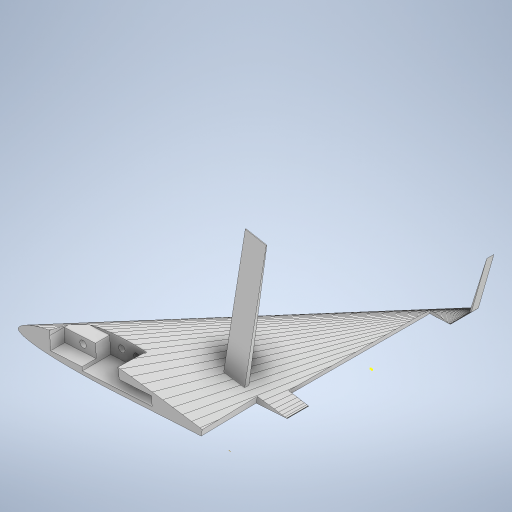
# Autodesk Inventor part: Część3
Saved by Autodesk Inventor 2023 (Build 270158000, 158)
## iProperties
Created: 2024-01-30
Part Number: Część3
Material: Ogólny
Document SubType Name: Modeling
Designer: domin
Density: 1 g/cm^3
Appearance: Domyślna
Author: domin
Autodesk Inventor part; units mm, degrees
ref_plane "YZ Plane" through (0, 0, 0) normal (1, 0, 0) x (0, 1, 0)
sketch "Szkic1" plane through (0, 0, 0) normal (0, 0, 1) x (1, 0, 0)
  line L0 (1, 0) -> (0.99647, 0.00045)
  line L1 (0.99647, 0.00045) -> (0.98625, 0.00202)
  line L2 (0.98625, 0.00202) -> (0.97011, 0.00489)
  line L3 (0.97011, 0.00489) -> (0.9487, 0.00881)
  line L4 (0.9487, 0.00881) -> (0.92238, 0.01337)
  line L5 (0.92238, 0.01337) -> (0.89128, 0.01841)
  line L6 (0.89128, 0.01841) -> (0.85576, 0.024)
  line L7 (0.85576, 0.024) -> (0.81633, 0.03011)
  line L8 (0.81633, 0.03011) -> (0.77357, 0.03666)
  line L9 (0.77357, 0.03666) -> (0.72806, 0.04352)
  line L10 (0.72806, 0.04352) -> (0.68043, 0.05055)
  line L11 (0.68043, 0.05055) -> (0.63132, 0.05759)
  line L12 (0.63132, 0.05759) -> (0.58139, 0.06441)
  line L13 (0.58139, 0.06441) -> (0.53129, 0.07079)
  line L14 (0.53129, 0.07079) -> (0.48169, 0.07638)
  line L15 (0.48169, 0.07638) -> (0.43306, 0.08075)
  line L16 (0.43306, 0.08075) -> (0.38567, 0.08362)
  line L17 (0.38567, 0.08362) -> (0.33981, 0.08483)
  line L18 (0.33981, 0.08483) -> (0.29573, 0.0843)
  line L19 (0.29573, 0.0843) -> (0.25363, 0.08205)
  line L20 (0.25363, 0.08205) -> (0.21371, 0.07819)
  line L21 (0.21371, 0.07819) -> (0.17625, 0.073)
  line L22 (0.17625, 0.073) -> (0.14162, 0.06669)
  line L23 (0.14162, 0.06669) -> (0.11018, 0.05944)
  line L24 (0.11018, 0.05944) -> (0.08225, 0.05143)
  line L25 (0.08225, 0.05143) -> (0.05808, 0.04282)
  line L26 (0.05808, 0.04282) -> (0.03791, 0.03383)
  line L27 (0.03791, 0.03383) -> (0.02189, 0.02468)
  line L28 (0.02189, 0.02468) -> (0.01015, 0.01565)
  line L29 (0.01015, 0.01565) -> (0.00279, 0.00714)
  line L30 (0.00279, 0.00714) -> (0, -0.00015)
  line L31 (0, -0.00015) -> (0.00304, -0.00626)
  line L32 (0.00304, -0.00626) -> (0.01212, -0.01204)
  line L33 (0.01212, -0.01204) -> (0.02628, -0.0175)
  line L34 (0.02628, -0.0175) -> (0.04543, -0.02234)
  line L35 (0.04543, -0.02234) -> (0.06943, -0.02649)
  line L36 (0.06943, -0.02649) -> (0.09807, -0.02991)
  line L37 (0.09807, -0.02991) -> (0.13109, -0.03257)
  line L38 (0.13109, -0.03257) -> (0.16817, -0.03448)
  line L39 (0.16817, -0.03448) -> (0.20893, -0.03565)
  line L40 (0.20893, -0.03565) -> (0.25292, -0.03611)
  line L41 (0.25292, -0.03611) -> (0.29966, -0.03586)
  line L42 (0.29966, -0.03586) -> (0.34861, -0.03487)
  line L43 (0.34861, -0.03487) -> (0.39937, -0.03302)
  line L44 (0.39937, -0.03302) -> (0.45165, -0.03044)
  line L45 (0.45165, -0.03044) -> (0.50495, -0.02744)
  line L46 (0.50495, -0.02744) -> (0.5586, -0.02425)
  line L47 (0.5586, -0.02425) -> (0.61189, -0.02102)
  line L48 (0.61189, -0.02102) -> (0.66414, -0.01787)
  line L49 (0.66414, -0.01787) -> (0.71467, -0.01488)
  line L50 (0.71467, -0.01488) -> (0.76283, -0.01212)
  line L51 (0.76283, -0.01212) -> (0.80796, -0.00963)
  line L52 (0.80796, -0.00963) -> (0.84948, -0.00744)
  line L53 (0.84948, -0.00744) -> (0.88681, -0.00555)
  line L54 (0.88681, -0.00555) -> (0.91942, -0.0039)
  line L55 (0.91942, -0.0039) -> (0.94699, -0.00239)
  line L56 (0.94699, -0.00239) -> (0.9693, -0.00108)
  line L57 (0.9693, -0.00108) -> (0.98598, -0.00026)
  line L58 (0.98598, -0.00026) -> (0.99643, 0)
  line L59 (0.99643, 0) -> (1, 0)
  point P0 (0, 0)
  dimension "d0" = 7.26481
  dimension "d1" = 178.531
  dimension "d2" = 8.69006
  dimension "d3" = 177.182
  dimension "d4" = 169.921
  dimension "d5" = 176.889
  dimension "d6" = 169.375
  dimension "d7" = 2.56425
  dimension "d8" = 169.6
  dimension "d9" = 1.94039
  dimension "d10" = 10.1614
  dimension "d11" = 1.67882
  dimension "d12" = 10.1632
  dimension "d13" = 1.54358
  dimension "d14" = 169.716
  dimension "d15" = 1.44409
  dimension "d16" = 169.577
  dimension "d17" = 1.3072
  dimension "d18" = 169.455
  dimension "d19" = 1.1312
  dimension "d20" = 169.349
  dimension "d21" = 0.89306
  dimension "d22" = 169.285
  dimension "d23" = 0.51316
  dimension "d24" = 169.267
  dimension "d25" = 0.00752
  dimension "d26" = 169.332
  dimension "d27" = 0.83462
  dimension "d28" = 169.514
  dimension "d29" = 2.12988
  dimension "d30" = 10.09
  dimension "d31" = 3.79914
  dimension "d32" = 9.35209
  dimension "d33" = 5.75343
  dimension "d34" = 8.42344
  dimension "d35" = 172.046
  dimension "d36" = 7.57127
  dimension "d37" = 169.676
  dimension "d38" = 167.212
  dimension "d39" = 6.6657
  dimension "d40" = 164.847
  dimension "d41" = 5.62061
  dimension "d42" = 162.409
  dimension "d43" = 4.3161
  dimension "d44" = 159.75
  dimension "d45" = 2.65917
  dimension "d46" = 156.733
  dimension "d47" = 0.45517
  dimension "d48" = 153.128
  dimension "d49" = 2.54557
  dimension "d50" = 148.712
  dimension "d51" = 6.91918
  dimension "d52" = 143.002
  dimension "d53" = 13.8215
  dimension "d54" = 135.169
  dimension "d55" = 25.2145
  dimension "d56" = 123.591
  dimension "d57" = 56.2828
  dimension "d58" = 103.678
  dimension "d59" = 0.12646
  dimension "d60" = 0
  dimension "d61" = 0.15175
  dimension "d62" = 0.02478
  dimension "d63" = 0.17465
  constraints: 120 end point, 1 horizontal
  measures "d0" angle of L0 L59
  measures "d1" angle of L0 L1
  measures "d2" angle of L0 L58
  measures "d3" angle of L0 L2
  measures "d4" angle of L0 L57
  measures "d5" angle of L0 L3
  measures "d6" angle of L0 L56
  measures "d7" angle of L0 L4
  measures "d8" angle of L0 L55
  measures "d9" angle of L0 L5
  measures "d10" angle of L0 L54
  measures "d11" angle of L0 L6
  measures "d12" angle of L0 L53
  measures "d13" angle of L0 L7
  measures "d14" angle of L0 L52
  measures "d15" angle of L0 L8
  measures "d16" angle of L0 L51
  measures "d17" angle of L0 L9
  measures "d18" angle of L0 L50
  measures "d19" angle of L0 L10
  measures "d20" angle of L0 L49
  measures "d21" angle of L0 L11
  measures "d22" angle of L0 L48
  measures "d23" angle of L0 L12
  measures "d24" angle of L0 L47
  measures "d25" angle of L0 L13
  measures "d26" angle of L0 L46
  measures "d27" angle of L0 L14
  measures "d28" angle of L0 L45
  measures "d29" angle of L0 L15
  measures "d30" angle of L0 L44
  measures "d31" angle of L0 L16
  measures "d32" angle of L0 L43
  measures "d33" angle of L0 L17
  measures "d34" angle of L0 L42
  measures "d35" angle of L0 L18
  measures "d36" angle of L0 L41
  measures "d37" angle of L0 L19
  measures "d38" angle of L0 L20
  measures "d39" angle of L0 L40
  measures "d40" angle of L0 L21
  measures "d41" angle of L0 L39
  measures "d42" angle of L0 L22
  measures "d43" angle of L0 L38
  measures "d44" angle of L0 L23
  measures "d45" angle of L0 L37
  measures "d46" angle of L0 L24
  measures "d47" angle of L0 L36
  measures "d48" angle of L0 L25
  measures "d49" angle of L0 L35
  measures "d50" angle of L0 L26
  measures "d51" angle of L0 L34
  measures "d52" angle of L0 L27
  measures "d53" angle of L0 L33
  measures "d54" angle of L0 L28
  measures "d55" angle of L0 L32
  measures "d56" angle of L0 L29
  measures "d57" angle of L0 L31
  measures "d58" angle of L0 L30
  measures "d59" distance from line of point (0, 0) L0
  measures "d60" distance from line of point (0, 0) L59
  measures "d61" distance from line of point (0, 0) L1
  measures "d62" distance from line of point (0, 0) L58
  measures "d63" distance from line of point (0, 0) L2
ref_plane "Płaszczyzna konstrukcyjna2" through (0, 0, 175) normal (0, 0, 1) x (1, 0, 0)
sketch "Szkic6" plane through (0, 0, 175) normal (0, 0, 1) x (1, 0, 0)
  line L0 (1, 0) -> (0.4705, 0.0675)
  line L1 (0.4705, 0.0675) -> (-1.0625, 0.303)
  line L2 (-1.0625, 0.303) -> (-3.4835, 0.7335)
  line L3 (-3.4835, 0.7335) -> (-6.695, 1.3215)
  line L4 (-6.695, 1.3215) -> (-10.643, 2.0055)
  line L5 (-10.643, 2.0055) -> (-15.308, 2.7615)
  line L6 (-15.308, 2.7615) -> (-20.636, 3.6)
  line L7 (-20.636, 3.6) -> (-26.5505, 4.5165)
  line L8 (-26.5505, 4.5165) -> (-32.9645, 5.499)
  line L9 (-32.9645, 5.499) -> (-39.791, 6.528)
  line L10 (-39.791, 6.528) -> (-46.9355, 7.5825)
  line L11 (-46.9355, 7.5825) -> (-54.302, 8.6385)
  line L12 (-54.302, 8.6385) -> (-61.7915, 9.6615)
  line L13 (-61.7915, 9.6615) -> (-69.3065, 10.6185)
  line L14 (-69.3065, 10.6185) -> (-76.7465, 11.457)
  line L15 (-76.7465, 11.457) -> (-84.041, 12.1125)
  line L16 (-84.041, 12.1125) -> (-91.1495, 12.543)
  line L17 (-91.1495, 12.543) -> (-98.0285, 12.7245)
  line L18 (-98.0285, 12.7245) -> (-104.6405, 12.645)
  line L19 (-104.6405, 12.645) -> (-110.9555, 12.3075)
  line L20 (-110.9555, 12.3075) -> (-116.9435, 11.7285)
  line L21 (-116.9435, 11.7285) -> (-122.5625, 10.95)
  line L22 (-122.5625, 10.95) -> (-127.757, 10.0035)
  line L23 (-127.757, 10.0035) -> (-132.473, 8.916)
  line L24 (-132.473, 8.916) -> (-136.6625, 7.7145)
  line L25 (-136.6625, 7.7145) -> (-140.288, 6.423)
  line L26 (-140.288, 6.423) -> (-143.3135, 5.0745)
  line L27 (-143.3135, 5.0745) -> (-145.7165, 3.702)
  line L28 (-145.7165, 3.702) -> (-147.4775, 2.3475)
  line L29 (-147.4775, 2.3475) -> (-148.5815, 1.071)
  line L30 (-148.5815, 1.071) -> (-149, -0.0225)
  line L31 (-149, -0.0225) -> (-148.544, -0.939)
  line L32 (-148.544, -0.939) -> (-147.182, -1.806)
  line L33 (-147.182, -1.806) -> (-145.058, -2.625)
  line L34 (-145.058, -2.625) -> (-142.1855, -3.351)
  line L35 (-142.1855, -3.351) -> (-138.5855, -3.9735)
  line L36 (-138.5855, -3.9735) -> (-134.2895, -4.4865)
  line L37 (-134.2895, -4.4865) -> (-129.3365, -4.8855)
  line L38 (-129.3365, -4.8855) -> (-123.7745, -5.172)
  line L39 (-123.7745, -5.172) -> (-117.6605, -5.3475)
  line L40 (-117.6605, -5.3475) -> (-111.062, -5.4165)
  line L41 (-111.062, -5.4165) -> (-104.051, -5.379)
  line L42 (-104.051, -5.379) -> (-96.7085, -5.2305)
  line L43 (-96.7085, -5.2305) -> (-89.0945, -4.953)
  line L44 (-89.0945, -4.953) -> (-81.2525, -4.566)
  line L45 (-81.2525, -4.566) -> (-73.2575, -4.116)
  line L46 (-73.2575, -4.116) -> (-65.21, -3.6375)
  line L47 (-65.21, -3.6375) -> (-57.2165, -3.153)
  line L48 (-57.2165, -3.153) -> (-49.379, -2.6805)
  line L49 (-49.379, -2.6805) -> (-41.7995, -2.232)
  line L50 (-41.7995, -2.232) -> (-34.5755, -1.818)
  line L51 (-34.5755, -1.818) -> (-27.806, -1.4445)
  line L52 (-27.806, -1.4445) -> (-21.578, -1.116)
  line L53 (-21.578, -1.116) -> (-15.9785, -0.8325)
  line L54 (-15.9785, -0.8325) -> (-11.087, -0.585)
  line L55 (-11.087, -0.585) -> (-6.9515, -0.3585)
  line L56 (-6.9515, -0.3585) -> (-3.605, -0.162)
  line L57 (-3.605, -0.162) -> (-1.103, -0.039)
  line L58 (-1.103, -0.039) -> (0.4645, 0)
  line L59 (0.4645, 0) -> (1, 0)
  point P0 (0, 0)
  dimension "d367" = 7.26481
  dimension "d368" = 178.531
  dimension "d369" = 8.69006
  dimension "d370" = 177.182
  dimension "d371" = 169.921
  dimension "d372" = 176.889
  dimension "d373" = 169.375
  dimension "d374" = 2.56425
  dimension "d375" = 169.6
  dimension "d376" = 1.94039
  dimension "d377" = 10.1614
  dimension "d378" = 1.67882
  dimension "d379" = 10.1632
  dimension "d380" = 1.54358
  dimension "d381" = 169.716
  dimension "d382" = 1.44409
  dimension "d383" = 169.577
  dimension "d384" = 1.3072
  dimension "d385" = 169.455
  dimension "d386" = 1.1312
  dimension "d387" = 169.349
  dimension "d388" = 0.89306
  dimension "d389" = 169.285
  dimension "d390" = 0.51316
  dimension "d391" = 169.267
  dimension "d392" = 0.00752
  dimension "d393" = 169.332
  dimension "d394" = 0.83462
  dimension "d395" = 169.514
  dimension "d396" = 2.12988
  dimension "d397" = 10.09
  dimension "d398" = 3.79914
  dimension "d399" = 9.35209
  dimension "d400" = 5.75343
  dimension "d401" = 8.42344
  dimension "d402" = 172.046
  dimension "d403" = 7.57127
  dimension "d404" = 169.676
  dimension "d405" = 167.212
  dimension "d406" = 6.6657
  dimension "d407" = 164.847
  dimension "d408" = 5.62061
  dimension "d409" = 162.409
  dimension "d410" = 4.3161
  dimension "d411" = 159.75
  dimension "d412" = 2.65917
  dimension "d413" = 156.733
  dimension "d414" = 0.45517
  dimension "d415" = 153.128
  dimension "d416" = 2.54557
  dimension "d417" = 148.712
  dimension "d418" = 6.91918
  dimension "d419" = 143.002
  dimension "d420" = 13.8215
  dimension "d421" = 135.169
  dimension "d422" = 25.2145
  dimension "d423" = 123.591
  dimension "d424" = 56.2828
  dimension "d425" = 103.678
  dimension "d426" = 0.12646
  dimension "d427" = 0
  dimension "d428" = 0.13816
  dimension "d429" = 0.01155
  dimension "d430" = 0.11231
  constraints: 120 end point, 1 horizontal
  measures "d367" angle of L0 L59
  measures "d368" angle of L0 L1
  measures "d369" angle of L0 L58
  measures "d370" angle of L0 L2
  measures "d371" angle of L0 L57
  measures "d372" angle of L0 L3
  measures "d373" angle of L0 L56
  measures "d374" angle of L0 L4
  measures "d375" angle of L0 L55
  measures "d376" angle of L0 L5
  measures "d377" angle of L0 L54
  measures "d378" angle of L0 L6
  measures "d379" angle of L0 L53
  measures "d380" angle of L0 L7
  measures "d381" angle of L0 L52
  measures "d382" angle of L0 L8
  measures "d383" angle of L0 L51
  measures "d384" angle of L0 L9
  measures "d385" angle of L0 L50
  measures "d386" angle of L0 L10
  measures "d387" angle of L0 L49
  measures "d388" angle of L0 L11
  measures "d389" angle of L0 L48
  measures "d390" angle of L0 L12
  measures "d391" angle of L0 L47
  measures "d392" angle of L0 L13
  measures "d393" angle of L0 L46
  measures "d394" angle of L0 L14
  measures "d395" angle of L0 L45
  measures "d396" angle of L0 L15
  measures "d397" angle of L0 L44
  measures "d398" angle of L0 L16
  measures "d399" angle of L0 L43
  measures "d400" angle of L0 L17
  measures "d401" angle of L0 L42
  measures "d402" angle of L0 L18
  measures "d403" angle of L0 L41
  measures "d404" angle of L0 L19
  measures "d405" angle of L0 L20
  measures "d406" angle of L0 L40
  measures "d407" angle of L0 L21
  measures "d408" angle of L0 L39
  measures "d409" angle of L0 L22
  measures "d410" angle of L0 L38
  measures "d411" angle of L0 L23
  measures "d412" angle of L0 L37
  measures "d413" angle of L0 L24
  measures "d414" angle of L0 L36
  measures "d415" angle of L0 L25
  measures "d416" angle of L0 L35
  measures "d417" angle of L0 L26
  measures "d418" angle of L0 L34
  measures "d419" angle of L0 L27
  measures "d420" angle of L0 L33
  measures "d421" angle of L0 L28
  measures "d422" angle of L0 L32
  measures "d423" angle of L0 L29
  measures "d424" angle of L0 L31
  measures "d425" angle of L0 L30
  measures "d426" distance from line of point (0, 0) L0
  measures "d427" distance from line of point (0, 0) L59
  measures "d428" distance from line of point (0, 0) L1
  measures "d429" distance from line of point (0, 0) L58
  measures "d430" distance from line of point (0, 0) L2
sketch "Szkic1 outline for Wyciągnięcie złożone2" plane through (0, 0, 0) normal (0, 0, 1) x (1, 0, 0)
  line L0 (0.98598, -0.00026) -> (0.99647, 0.00045)
  line L1 (0.9693, -0.00108) -> (0.98598, -0.00026)
  line L2 (0.94699, -0.00239) -> (0.9693, -0.00108)
  line L3 (0.91942, -0.0039) -> (0.94699, -0.00239)
  line L4 (0.88681, -0.00555) -> (0.91942, -0.0039)
  line L5 (0.84948, -0.00744) -> (0.88681, -0.00555)
  line L6 (0.80796, -0.00963) -> (0.84948, -0.00744)
  line L7 (0.76283, -0.01212) -> (0.80796, -0.00963)
  line L8 (0.71467, -0.01488) -> (0.76283, -0.01212)
  line L9 (0.66414, -0.01787) -> (0.71467, -0.01488)
  line L10 (0.61189, -0.02102) -> (0.66414, -0.01787)
  line L11 (0.5586, -0.02425) -> (0.61189, -0.02102)
  line L12 (0.50495, -0.02744) -> (0.5586, -0.02425)
  line L13 (0.45165, -0.03044) -> (0.50495, -0.02744)
  line L14 (0.39937, -0.03302) -> (0.45165, -0.03044)
  line L15 (0.34861, -0.03487) -> (0.39937, -0.03302)
  line L16 (0.29966, -0.03586) -> (0.34861, -0.03487)
  line L17 (0.25292, -0.03611) -> (0.29966, -0.03586)
  line L18 (0.20893, -0.03565) -> (0.25292, -0.03611)
  line L19 (0.16817, -0.03448) -> (0.20893, -0.03565)
  line L20 (0.13109, -0.03257) -> (0.16817, -0.03448)
  line L21 (0.09807, -0.02991) -> (0.13109, -0.03257)
  line L22 (0.06943, -0.02649) -> (0.09807, -0.02991)
  line L23 (0.04543, -0.02234) -> (0.06943, -0.02649)
  line L24 (0.02628, -0.0175) -> (0.04543, -0.02234)
  line L25 (0.01212, -0.01204) -> (0.02628, -0.0175)
  line L26 (0.00304, -0.00626) -> (0.01212, -0.01204)
  line L27 (0, -0.00015) -> (0.00304, -0.00626)
  line L28 (0.00279, 0.00714) -> (0, -0.00015)
  line L29 (0.01015, 0.01565) -> (0.00279, 0.00714)
  line L30 (0.02189, 0.02468) -> (0.01015, 0.01565)
  line L31 (0.03791, 0.03383) -> (0.02189, 0.02468)
  line L32 (0.05808, 0.04282) -> (0.03791, 0.03383)
  line L33 (0.08225, 0.05143) -> (0.05808, 0.04282)
  line L34 (0.11018, 0.05944) -> (0.08225, 0.05143)
  line L35 (0.14162, 0.06669) -> (0.11018, 0.05944)
  line L36 (0.17625, 0.073) -> (0.14162, 0.06669)
  line L37 (0.21371, 0.07819) -> (0.17625, 0.073)
  line L38 (0.25363, 0.08205) -> (0.21371, 0.07819)
  line L39 (0.29573, 0.0843) -> (0.25363, 0.08205)
  line L40 (0.33981, 0.08483) -> (0.29573, 0.0843)
  line L41 (0.38567, 0.08362) -> (0.33981, 0.08483)
  line L42 (0.43306, 0.08075) -> (0.38567, 0.08362)
  line L43 (0.48169, 0.07638) -> (0.43306, 0.08075)
  line L44 (0.53129, 0.07079) -> (0.48169, 0.07638)
  line L45 (0.58139, 0.06441) -> (0.53129, 0.07079)
  line L46 (0.63132, 0.05759) -> (0.58139, 0.06441)
  line L47 (0.68043, 0.05055) -> (0.63132, 0.05759)
  line L48 (0.72806, 0.04352) -> (0.68043, 0.05055)
  line L49 (0.77357, 0.03666) -> (0.72806, 0.04352)
  line L50 (0.81633, 0.03011) -> (0.77357, 0.03666)
  line L51 (0.85576, 0.024) -> (0.81633, 0.03011)
  line L52 (0.89128, 0.01841) -> (0.85576, 0.024)
  line L53 (0.92238, 0.01337) -> (0.89128, 0.01841)
  line L54 (0.9487, 0.00881) -> (0.92238, 0.01337)
  line L55 (0.97011, 0.00489) -> (0.9487, 0.00881)
  line L56 (0.98625, 0.00202) -> (0.97011, 0.00489)
  line L57 (0.99647, 0.00045) -> (0.98625, 0.00202)
sketch "Szkic6 outline for Wyciągnięcie złożone2" plane through (0, 0, 175) normal (0, 0, 1) x (1, 0, 0)
  line L0 (0.4645, 0) -> (1, 0)
  line L1 (-1.103, -0.039) -> (0.4645, 0)
  line L2 (-3.605, -0.162) -> (-1.103, -0.039)
  line L3 (-6.9515, -0.3585) -> (-3.605, -0.162)
  line L4 (-11.087, -0.585) -> (-6.9515, -0.3585)
  line L5 (-15.9785, -0.8325) -> (-11.087, -0.585)
  line L6 (-21.578, -1.116) -> (-15.9785, -0.8325)
  line L7 (-27.806, -1.4445) -> (-21.578, -1.116)
  line L8 (-34.5755, -1.818) -> (-27.806, -1.4445)
  line L9 (-41.7995, -2.232) -> (-34.5755, -1.818)
  line L10 (-49.379, -2.6805) -> (-41.7995, -2.232)
  line L11 (-57.2165, -3.153) -> (-49.379, -2.6805)
  line L12 (-65.21, -3.6375) -> (-57.2165, -3.153)
  line L13 (-73.2575, -4.116) -> (-65.21, -3.6375)
  line L14 (-81.2525, -4.566) -> (-73.2575, -4.116)
  line L15 (-89.0945, -4.953) -> (-81.2525, -4.566)
  line L16 (-96.7085, -5.2305) -> (-89.0945, -4.953)
  line L17 (-104.051, -5.379) -> (-96.7085, -5.2305)
  line L18 (-111.062, -5.4165) -> (-104.051, -5.379)
  line L19 (-117.6605, -5.3475) -> (-111.062, -5.4165)
  line L20 (-123.7745, -5.172) -> (-117.6605, -5.3475)
  line L21 (-129.3365, -4.8855) -> (-123.7745, -5.172)
  line L22 (-134.2895, -4.4865) -> (-129.3365, -4.8855)
  line L23 (-138.5855, -3.9735) -> (-134.2895, -4.4865)
  line L24 (-142.1855, -3.351) -> (-138.5855, -3.9735)
  line L25 (-145.058, -2.625) -> (-142.1855, -3.351)
  line L26 (-147.182, -1.806) -> (-145.058, -2.625)
  line L27 (-148.544, -0.939) -> (-147.182, -1.806)
  line L28 (-149, -0.0225) -> (-148.544, -0.939)
  line L29 (-148.5815, 1.071) -> (-149, -0.0225)
  line L30 (-147.4775, 2.3475) -> (-148.5815, 1.071)
  line L31 (-145.7165, 3.702) -> (-147.4775, 2.3475)
  line L32 (-143.3135, 5.0745) -> (-145.7165, 3.702)
  line L33 (-140.288, 6.423) -> (-143.3135, 5.0745)
  line L34 (-136.6625, 7.7145) -> (-140.288, 6.423)
  line L35 (-132.473, 8.916) -> (-136.6625, 7.7145)
  line L36 (-127.757, 10.0035) -> (-132.473, 8.916)
  line L37 (-122.5625, 10.95) -> (-127.757, 10.0035)
  line L38 (-116.9435, 11.7285) -> (-122.5625, 10.95)
  line L39 (-110.9555, 12.3075) -> (-116.9435, 11.7285)
  line L40 (-104.6405, 12.645) -> (-110.9555, 12.3075)
  line L41 (-98.0285, 12.7245) -> (-104.6405, 12.645)
  line L42 (-91.1495, 12.543) -> (-98.0285, 12.7245)
  line L43 (-84.041, 12.1125) -> (-91.1495, 12.543)
  line L44 (-76.7465, 11.457) -> (-84.041, 12.1125)
  line L45 (-69.3065, 10.6185) -> (-76.7465, 11.457)
  line L46 (-61.7915, 9.6615) -> (-69.3065, 10.6185)
  line L47 (-54.302, 8.6385) -> (-61.7915, 9.6615)
  line L48 (-46.9355, 7.5825) -> (-54.302, 8.6385)
  line L49 (-39.791, 6.528) -> (-46.9355, 7.5825)
  line L50 (-32.9645, 5.499) -> (-39.791, 6.528)
  line L51 (-26.5505, 4.5165) -> (-32.9645, 5.499)
  line L52 (-20.636, 3.6) -> (-26.5505, 4.5165)
  line L53 (-15.308, 2.7615) -> (-20.636, 3.6)
  line L54 (-10.643, 2.0055) -> (-15.308, 2.7615)
  line L55 (-6.695, 1.3215) -> (-10.643, 2.0055)
  line L56 (-3.4835, 0.7335) -> (-6.695, 1.3215)
  line L57 (-1.0625, 0.303) -> (-3.4835, 0.7335)
  line L58 (0.4705, 0.0675) -> (-1.0625, 0.303)
  line L59 (1, 0) -> (0.4705, 0.0675)
loft "Wyciągnięcie złożone2" add profiles "Szkic1 outline for Wyciągnięcie złożone2", "Szkic6 outline for Wyciągnięcie złożone2"
ref_plane "Płaszczyzna konstrukcyjna3" through (0.48169, 0.07638, 0) normal (0.1803699, 0.9834745, 0.0156405) x (-0.4030251, 0.0593912, 0.9132598)
sketch "Szkic7" plane through (0.48169, 0.07638, 0) normal (0.1803699, 0.9834745, 0.0156405) x (-0.4030251, 0.0593912, 0.9132598)
  point P0 (0.189597, -0.419128)
sketch "Szkic8" plane through (0.48169, 0.07638, 0) normal (0.1803699, 0.9834745, 0.0156405) x (-0.4030251, 0.0593912, 0.9132598)
  line L0 (-0.213428, 0.478111) -> (159.607033, 71.716644)
  line L1 (159.296463, 72.413394) -> (123.078817, 55.43452)
  line L2 (123.078817, 55.43452) -> (131.97543, 36.457148)
  line L3 (131.97543, 36.457148) -> (168.193076, 53.436022)
  line L4 (168.193076, 53.436022) -> (159.296463, 72.413394)
  point P0 (0.189597, -0.419128)
  dimension "d493" = 40
  dimension "d494" = 91.0927
  dimension "d495" = 20.95926
  dimension "d496" = 0.01455
  constraints: 8 end point, 2 parallel, 1 perpendicular, 1 point on line
  measures "d493" distance of L1.start L1.end
  measures "d494" angle of L4 L0
  measures "d495" distance between parallel lines of L1 L3
  measures "d496" distance from line of L0.end L4
sketch "Szkic8 outline for Wyciągnięcie proste2" plane through (0.48169, 0.07638, 0) normal (0.1803699, 0.9834745, 0.0156405) x (-0.4030251, 0.0593912, 0.9132598)
  line L0 (168.193076, 53.436022) -> (159.296463, 72.413394)
  line L1 (131.97543, 36.457148) -> (168.193076, 53.436022)
  line L2 (123.078817, 55.43452) -> (131.97543, 36.457148)
  line L3 (159.296463, 72.413394) -> (123.078817, 55.43452)
extrude "Wyciągnięcie proste2" cut sketch "Szkic8 outline for Wyciągnięcie proste2" along normal blind 40 and the other way blind 5
sketch "Szkic9" plane through (0.48169, 0.07638, 0) normal (0.1803699, 0.9834745, 0.0156405) x (-0.4030251, 0.0593912, 0.9132598)
  line L0 (-0.207793, 0.465576) -> (123.755437, 53.991221)
  line L1 (109.292588, 48.877352) -> (17.90185, 8.285075)
  line L2 (17.90185, 8.285075) -> (23.584769, -4.509628)
  line L3 (23.584769, -4.509628) -> (114.975507, 36.082648)
  line L4 (114.975507, 36.082648) -> (109.292588, 48.877352)
  line L5 (-0.207767, 0.465428) -> (123.16026, 55.260795)
  point P0 (0.189597, -0.419128)
  dimension "d501" = 100
  dimension "d502" = 14
  dimension "d503" = 14.20467
  constraints: 8 end point, 3 parallel, 1 perpendicular, 1 point on line
  measures "d501" distance of L1.start L1.end
  measures "d502" distance of L2.end L1.end
  measures "d503" distance between parallel lines of L3 L5
sketch "Szkic9 outline for Wyciągnięcie proste3" plane through (0.48169, 0.07638, 0) normal (0.1803699, 0.9834745, 0.0156405) x (-0.4030251, 0.0593912, 0.9132598)
  line L0 (23.584769, -4.509628) -> (114.975507, 36.082648)
  line L1 (17.90185, 8.285075) -> (23.584769, -4.509628)
  line L2 (109.292588, 48.877352) -> (17.90185, 8.285075)
  line L3 (114.975507, 36.082648) -> (109.292588, 48.877352)
extrude "Wyciągnięcie proste3" cut sketch "Szkic9 outline for Wyciągnięcie proste3" along normal mid plane 40
sketch "Szkic10" plane through (0.75051, -0.004627, 19.726044) normal (-0.9835902, 0.1804121, -0.001318) x (-0.0013322, 0.0000425, 0.9999991)
  line L0 (-0.001049, -1.278668) -> (-0.001049, 2.727934)
  line L1 (-0.001049, 2.727934) -> (100.015608, 2.727934)
  line L2 (100.015608, 2.727934) -> (100.015608, -1.278668)
  line L3 (100.015608, -1.278668) -> (-0.001049, -1.278668)
  point P0 (-19.725026, -0.134767)
  dimension "d506" = 100.01666
  dimension "d507" = 4.0066
  dimension "d508" = 119.74063
  dimension "d509" = 2.8627
  constraints: 8 end point, 2 parallel, 1 perpendicular, 1 vertical
  measures "d506" distance between parallel lines of L0 L2
  measures "d507" distance between parallel lines of L1 L3
  measures "d508" distance from line of point (-19.725, -0.135) L2
  measures "d509" distance from line of point (-19.725, -0.135) L1
sketch "Szkic10 outline for Wyciągnięcie proste4" plane through (0.75051, -0.004627, 19.726044) normal (-0.9835902, 0.1804121, -0.001318) x (-0.0013322, 0.0000425, 0.9999991)
  line L0 (-0.001049, -1.278668) -> (100.015608, -1.278668)
  line L1 (-0.001049, 2.727934) -> (-0.001049, -1.278668)
  line L2 (100.015608, 2.727934) -> (-0.001049, 2.727934)
  line L3 (100.015608, -1.278668) -> (100.015608, 2.727934)
extrude "Wyciągnięcie proste4" cut sketch "Szkic10 outline for Wyciągnięcie proste4" against normal blind 40
sketch "Szkic11" plane through (0.48169, 0.07638, 0) normal (0.1803699, 0.9834745, 0.0156405) x (-0.4030251, 0.0593912, 0.9132598)
  line L0 (135.985358, 29.037386) -> (142.052879, 15.319325)
  line L1 (142.052879, 15.319325) -> (139.271225, 14.088995)
  line L2 (139.271225, 14.088995) -> (133.203705, 27.807056)
  line L3 (133.203705, 27.807056) -> (135.985358, 29.037386)
  line L4 (109.294392, 48.880488) -> (123.256327, 55.055874)
  point P0 (0.189597, -0.419128)
  dimension "d512" = 15
  dimension "d513" = 43.94379
  dimension "d514" = 3.0416
  dimension "d515" = 1.11666
  constraints: 8 end point, 3 parallel, 1 perpendicular
  measures "d512" distance of L0.start L0.end
  measures "d513" distance between parallel lines of L1 L4
  measures "d514" distance between parallel lines of L2 L0
  measures "d515" distance from line of L4.end L0
ref_plane "Płaszczyzna konstrukcyjna4" through (14.911285, 78.754339, 1.251243) normal (0.1803699, 0.9834745, 0.0156405) x (-0.4030251, 0.0593912, 0.9132598)
sketch "Szkic12" plane through (14.911285, 78.754339, 1.251243) normal (0.1803699, 0.9834745, 0.0156405) x (-0.4030251, 0.0593912, 0.9132598)
  line L0 (127.002296, 9.641147) -> (133.116013, -4.056388)
  line L1 (133.116013, -4.056388) -> (132.659429, -4.260179)
  line L2 (132.659429, -4.260179) -> (126.545711, 9.437356)
  line L3 (126.545711, 9.437356) -> (127.002296, 9.641147)
  line L4 (173.622172, 40.301894) -> (176.434537, 34.000905)
  point P0 (0.189597, -0.419128)
  dimension "d517" = 15
  dimension "d518" = 0.5
  dimension "d519" = 55.06857
  dimension "d520" = 17.09693
  constraints: 8 end point, 3 parallel, 1 perpendicular
  measures "d517" distance of L0.start L0.end
  measures "d518" distance of L0.end L1.end
  measures "d519" distance between parallel lines of L0 L4
  measures "d520" distance from line of L4.end L1
sketch "Szkic11 outline for Wyciągnięcie złożone3" plane through (0.48169, 0.07638, 0) normal (0.1803699, 0.9834745, 0.0156405) x (-0.4030251, 0.0593912, 0.9132598)
  line L0 (135.985358, 29.037386) -> (142.052879, 15.319325)
  line L1 (142.052879, 15.319325) -> (139.271225, 14.088995)
  line L2 (139.271225, 14.088995) -> (133.203705, 27.807056)
  line L3 (133.203705, 27.807056) -> (135.985358, 29.037386)
sketch "Szkic12 outline for Wyciągnięcie złożone3" plane through (14.911285, 78.754339, 1.251243) normal (0.1803699, 0.9834745, 0.0156405) x (-0.4030251, 0.0593912, 0.9132598)
  line L0 (127.002296, 9.641147) -> (133.116013, -4.056388)
  line L1 (133.116013, -4.056388) -> (132.659429, -4.260179)
  line L2 (132.659429, -4.260179) -> (126.545711, 9.437356)
  line L3 (126.545711, 9.437356) -> (127.002296, 9.641147)
loft "Wyciągnięcie złożone3" add profiles "Szkic11 outline for Wyciągnięcie złożone3", "Szkic12 outline for Wyciągnięcie złożone3"
ref_plane "Płaszczyzna konstrukcyjna5" through (-73.2575, -4.116, 75) normal (0, 0, 1) x (0.998237, 0.0593546, 0)
sketch "Szkic13" plane through (-73.2575, -4.116, 75) normal (0, 0, 1) x (0.998237, 0.0593546, 0)
  point P0 (74.370885, -0.298783)
  point P1 (73.372639, -0.239578)
sketch "Szkic14" plane through (0.5586, -0.02425, 0) normal (0, 0, -1) x (-0.998237, -0.0593546, 0)
  line L0 (-0.442061, -0.001992) -> (-0.028848, 0.022578)
  line L1 (-0.442061, -0.001992) -> (-13.747584, 37.720191)
  line L2 (-13.747584, 37.720191) -> (0.556176, 0.057363)
  line L3 (0.556176, 0.057363) -> (-0.442061, -0.001992)
  point P0 (-0.028848, 0.022578)
  dimension "d529" = 40
  dimension "d530" = 72.6068
  constraints: 6 end point
  measures "d529" distance of L0.start L1.end
  measures "d530" angle of L0 L2
sketch "Szkic14 outline for Wyciągnięcie proste5" plane through (0.5586, -0.02425, 0) normal (0, 0, -1) x (-0.998237, -0.0593546, 0)
  line L0 (0.556176, 0.057363) -> (-13.747584, 37.720191)
  line L1 (-0.028848, 0.022578) -> (0.556176, 0.057363)
  line L2 (-0.442061, -0.001992) -> (-0.028848, 0.022578)
  line L3 (-13.747584, 37.720191) -> (-0.442061, -0.001992)
extrude "Wyciągnięcie proste5" add sketch "Szkic14 outline for Wyciągnięcie proste5" against normal blind 5
sketch "Szkic15" plane through (-73.2575, -4.116, 175) normal (0, 0, 1) x (0.998237, 0.0593546, 0)
  line L0 (73.393138, -0.185477) -> (-62.591019, 15.573023)
  line L1 (-52.57508, 14.412327) -> (-26.178063, 14.412327)
  line L2 (-26.178063, 14.412327) -> (-26.178063, 5.251261)
  line L3 (-26.178063, 5.251261) -> (-52.57508, 5.251261)
  line L4 (-52.57508, 5.251261) -> (-52.57508, 14.412327)
  line L5 (73.404728, -0.154958) -> (-48.323836, 17.965918)
  line L6 (-30.254483, 15.27606) -> (-3.85609, 15.27606)
  line L7 (-3.85609, 15.27606) -> (-3.85609, 2.834354)
  line L8 (-3.85609, 2.834354) -> (-30.254483, 2.834354)
  line L9 (-30.254483, 2.834354) -> (-30.254483, 15.27606)
  line L10 (-3.85609, 9.055207) -> (19.099741, 9.055207)
  line L11 (19.099741, 9.055207) -> (19.099741, 2.834354)
  line L12 (19.099741, 2.834354) -> (-3.85609, 2.834354)
  line L13 (-3.85609, 2.834354) -> (-3.85609, 9.055207)
  point P0 (73.372648, -0.239428)
  point P1 (-3.85609, 2.834354)
  dimension "d533" = 22.95583
  dimension "d534" = 45.2778
  dimension "d535" = 49.35422
  dimension "d536" = 71.67482
  dimension "d537" = 6.22085
  dimension "d538" = 5.35712
  dimension "d539" = 3.80395
  constraints: 24 end point, 6 parallel, 3 horizontal, 3 perpendicular, 3 point on line, 1 midpoint
  measures "d533" distance between parallel lines of L11 L7
  measures "d534" distance between parallel lines of L11 L2
  measures "d535" distance between parallel lines of L9 L11
  measures "d536" distance between parallel lines of L11 L4
  measures "d537" distance between parallel lines of L10 L8
  measures "d538" distance between parallel lines of L10 L1
  measures "d539" distance between parallel lines of L10 L3
sketch "Szkic15 outline for Wyciągnięcie proste6" plane through (-73.2575, -4.116, 175) normal (0, 0, 1) x (0.998237, 0.0593546, 0)
  line L0 (-26.178063, 5.251261) -> (-26.178063, 14.412327)
  line L1 (-52.57508, 5.251261) -> (-26.178063, 5.251261)
  line L2 (-52.57508, 14.412327) -> (-52.57508, 5.251261)
  line L3 (-26.178063, 14.412327) -> (-52.57508, 14.412327)
extrude "Wyciągnięcie proste6" cut sketch "Szkic15 outline for Wyciągnięcie proste6" against normal blind 10
sketch "Szkic15 outline for Wyciągnięcie proste7" plane through (-73.2575, -4.116, 175) normal (0, 0, 1) x (0.998237, 0.0593546, 0)
  line L0 (-30.254483, 2.834354) -> (-3.85609, 2.834354)
  line L1 (-30.254483, 15.27606) -> (-30.254483, 2.834354)
  line L2 (-3.85609, 15.27606) -> (-30.254483, 15.27606)
  line L3 (-3.85609, 2.834354) -> (-3.85609, 15.27606)
extrude "Wyciągnięcie proste7" cut sketch "Szkic15 outline for Wyciągnięcie proste7" against normal blind 20
sketch "Szkic15 outline for Wyciągnięcie proste8" plane through (-73.2575, -4.116, 175) normal (0, 0, 1) x (0.998237, 0.0593546, 0)
  line L0 (-3.85609, 2.834354) -> (19.099741, 2.834354)
  line L1 (-3.85609, 9.055207) -> (-3.85609, 2.834354)
  line L2 (19.099741, 9.055207) -> (-3.85609, 9.055207)
  line L3 (19.099741, 2.834354) -> (19.099741, 9.055207)
extrude "Wyciągnięcie proste8" cut sketch "Szkic15 outline for Wyciągnięcie proste8" against normal blind 20
sketch "Szkic16" plane through (-73.2575, -4.116, 175) normal (0, 0, 1) x (0.998237, 0.0593546, 0)
  line L0 (73.393138, -0.185477) -> (-62.591019, 15.573023)
  line L1 (-52.445785, 14.397344) -> (-4.400631, 14.397344)
  line L2 (-4.400631, 14.397344) -> (-4.400631, 23.16966)
  line L3 (-4.400631, 23.16966) -> (-52.445785, 23.16966)
  line L4 (-52.445785, 23.16966) -> (-52.445785, 14.397344)
  point P0 (73.372648, -0.239428)
  dimension "d546" = 48.04515
  dimension "d547" = 8.77232
  dimension "d548" = 77.79377
  constraints: 8 end point, 2 parallel, 1 horizontal, 1 perpendicular, 1 point on line
  measures "d546" distance between parallel lines of L2 L4
  measures "d547" distance between parallel lines of L1 L3
  measures "d548" distance from line of L0.start L2
sketch "Szkic16 outline for Wyciągnięcie proste9" plane through (-73.2575, -4.116, 175) normal (0, 0, 1) x (0.998237, 0.0593546, 0)
  line L0 (-4.400631, 23.16966) -> (-52.445785, 23.16966)
  line L1 (-4.400631, 14.397344) -> (-4.400631, 23.16966)
  line L2 (-52.445785, 14.397344) -> (-4.400631, 14.397344)
  line L3 (-52.445785, 23.16966) -> (-52.445785, 14.397344)
extrude "Wyciągnięcie proste9" cut sketch "Szkic16 outline for Wyciągnięcie proste9" against normal blind 20
sketch "Szkic17" plane through (-73.2575, -4.116, 165) normal (0, 0, 1) x (0.998237, 0.0593546, 0)
  point P0 (73.372648, -0.239428)
  point P1 (-39.303704, 10.023918)
hole "Otwór1" at (-113.086876, 3.557388, 165) direction (0, 0, -1) diameter 4.5 depth 8 tip angle 118 clearance for "Śruba ze łbem stożkowym ISO 2009/7046" size "M4" standard "ISO"
sketch "Szkic18" plane through (-73.2575, -4.116, 155) normal (0, 0, 1) x (0.998237, 0.0593546, 0)
  point P0 (73.372648, -0.239428)
  point P1 (-21.927849, 9.730808)
  point P2 (-11.27743, 9.463991)
hole "Otwór2" at (-95.724257, 4.296133, 155) at (-85.076779, 4.661938, 155) direction (0, 0, -1) diameter 4.5 depth 8 tip angle 118 clearance for "Wkręt z łbem walcowym z rowkiem ISO 1207" size "M4" standard "ISO"
